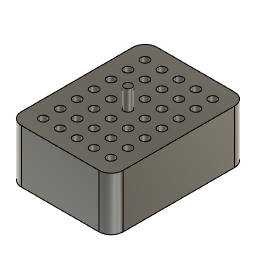
Blade Holder v2 (Autodesk Fusion 360 design; units mm, degrees)
Autodesk Fusion 360 part; units mm, degrees
sketch "Sketch1" plane through (0, 0, 0) normal (0, 0, 1) x (1, 0, 0) in component "Blades"
  circle A0 centre (0, 0) radius 1.595
  dimension "d1" = 3.19
  constraint coincident A0.centre origin
  measures "d1" diameter of A0
extrude "Extrude1" add sketch "Sketch1" along normal blind 28.3 makes body 1 in component "Blades"
sketch "Sketch1 (2)" plane through (0, 0, 0) normal (0, 0, 1) x (1, 0, 0) in component "Holder"
  circle A0 centre (0, 0) radius 1.72
  circle A1 centre (-14, -21) radius 1.72
  circle A2 centre (-7, -21) radius 1.72
  circle A3 centre (-14, -14) radius 1.72
  circle A4 centre (-7, -14) radius 1.72
  circle A5 centre (-14, -7) radius 1.72
  line L0 (-21, -28) -> (21, -28)
  line L1 (21, -28) -> (21, 28)
  line L2 (21, 28) -> (-21, 28)
  line L3 (-21, 28) -> (-21, -28)
  circle A6 centre (0, -21) radius 1.72
  circle A7 centre (7, -21) radius 1.72
  circle A8 centre (14, -21) radius 1.72
  circle A9 centre (0, -14) radius 1.72
  circle A10 centre (7, -14) radius 1.72
  circle A11 centre (14, -14) radius 1.72
  circle A12 centre (-7, -7) radius 1.72
  circle A13 centre (0, -7) radius 1.72
  circle A14 centre (7, -7) radius 1.72
  circle A15 centre (14, -7) radius 1.72
  circle A16 centre (-14, 0) radius 1.72
  circle A17 centre (-7, 0) radius 1.72
  circle A18 centre (7, 0) radius 1.72
  circle A19 centre (14, 0) radius 1.72
  circle A20 centre (-14, 7) radius 1.72
  circle A21 centre (-7, 7) radius 1.72
  circle A22 centre (0, 7) radius 1.72
  circle A23 centre (7, 7) radius 1.72
  circle A24 centre (14, 7) radius 1.72
  circle A25 centre (-14, 14) radius 1.72
  circle A26 centre (-7, 14) radius 1.72
  circle A27 centre (0, 14) radius 1.72
  circle A28 centre (7, 14) radius 1.72
  circle A29 centre (14, 14) radius 1.72
  circle A30 centre (-14, 21) radius 1.72
  circle A31 centre (-7, 21) radius 1.72
  circle A32 centre (0, 21) radius 1.72
  circle A33 centre (7, 21) radius 1.72
  circle A34 centre (14, 21) radius 1.72
  line L4 (21, 0) -> (0, 0) construction
  line L5 (0, 0) -> (0, 28) construction
  dimension "d8" = 7
  dimension "d9" = 7
  dimension "d12" = 3.44
  dimension "d24" = 42
  dimension "d25" = 56
  constraint horizontal L0
  constraint vertical L1
  constraint horizontal L2
  constraint vertical L3
  constraint coincident A0.centre L4.end
  constraint midpoint L1 L4.start
  constraint midpoint L2 L5.end
  constraint perpendicular L2 L5
  constraint perpendicular L1 L4
  measures "d12" diameter of A0
  measures "d24" distance of L1 L3
  measures "d25" distance of L0.end L1.end
extrude "Extrude1'" add sketch "Sketch1 (2)" along normal blind 20 separate body makes body 2 in component "Holder"
sketch "Sketch2" plane through (0, 0, 0) normal (0, 0, -1) x (1, 0, 0) in component "Holder"
  circle A0 centre (-7, -7) radius 1.72 construction
  circle A1 centre (-14, -7) radius 1.72 construction
  circle A2 centre (14, 0) radius 1.72 construction
  circle A3 centre (7, 0) radius 1.72 construction
  circle A4 centre (-7, 0) radius 1.72 construction
  circle A5 centre (7, 14) radius 1.72 construction
  circle A6 centre (14, 14) radius 1.72 construction
  circle A7 centre (-7, 7) radius 1.72 construction
  circle A8 centre (0, 7) radius 1.72 construction
  circle A9 centre (7, 7) radius 1.72 construction
  circle A10 centre (-14, 0) radius 1.72 construction
  circle A11 centre (14, 7) radius 1.72 construction
  circle A12 centre (0, 14) radius 1.72 construction
  circle A13 centre (0, -7) radius 1.72 construction
  circle A14 centre (7, -7) radius 1.72 construction
  circle A15 centre (14, -7) radius 1.72 construction
  circle A16 centre (-14, -14) radius 1.72 construction
  circle A17 centre (-7, -14) radius 1.72 construction
  circle A18 centre (0, -14) radius 1.72 construction
  circle A19 centre (7, -14) radius 1.72 construction
  circle A20 centre (14, -14) radius 1.72 construction
  circle A21 centre (-14, -21) radius 1.72 construction
  circle A22 centre (-7, -21) radius 1.72 construction
  circle A23 centre (0, -21) radius 1.72 construction
  circle A24 centre (7, -21) radius 1.72 construction
  circle A25 centre (14, -21) radius 1.72 construction
  circle A26 centre (7, 21) radius 1.72 construction
  circle A27 centre (-14, 21) radius 1.72 construction
  circle A28 centre (14, 21) radius 1.72 construction
  circle A29 centre (0, 21) radius 1.72 construction
  circle A30 centre (0, 0) radius 1.72 construction
  circle A31 centre (-7, 21) radius 1.72 construction
  circle A32 centre (-7, 14) radius 1.72 construction
  circle A33 centre (-14, 14) radius 1.72 construction
  circle A34 centre (-14, 7) radius 1.72 construction
  line L0 (-21, 28) -> (-21, -28)
  line L1 (-21, -28) -> (21, -28)
  line L2 (21, -28) -> (21, 28)
  line L3 (21, 28) -> (-21, 28)
extrude "Extrude2" add sketch "Sketch2" along normal blind 2 bodies 2 in component "Holder"
fillet "Fillet2" radius 5 4 edges at (-21, -28, 9) (21, -28, 9) (-21, 28, 9) (21, 28, 9) on bodies 2 in component "Holder"
component "Blades" placed x (1, 0, 0) y (0, 1, 0) z (0, 0, 1) at (0, 0, 0)
component "Holder" placed x (1, 0, 0) y (0, 1, 0) z (0, 0, 1) at (0, 0, 0)
equation "d1 = blade_shaft_diameter"
equation "rows = 5"
equation "columns = 7"
equation "d6 = rows"
equation "d7 = columns"
equation "d8 = spacing"
equation "d9 = spacing"
equation "blade_shaft_diameter = 3.19 mm"
equation "blade_shaft_clearance = 0.25 mm"
equation "d12 = blade_shaft_diameter + blade_shaft_clearance"
equation "spacing = 7 mm"
equation "d24 = spacing * ( rows + 1 )"
equation "d25 = spacing * ( columns + 1 )"
